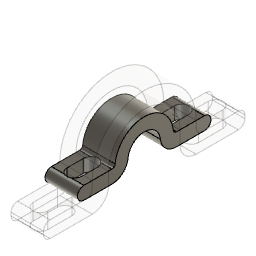
spiral_sleve_holders (Autodesk Fusion 360 design; units mm, degrees)
Autodesk Fusion 360 part; units mm, degrees
sketch "Sketch1" plane through (0, 0, 0) normal (1, 0, 0) x (0, 1, 0) in component "small_spiral_sleve_holder"
  circle A0 centre (0, 0) radius 5
  circle A1 centre (0, 0) radius 9
  line L0 (0, 0) -> (0, -5) construction
  line L1 (8.0623, -4) -> (20.5623, -4)
  line L2 (20.5623, -4) -> (20.5623, 0)
  line L3 (20.5623, 0) -> (9, 0)
  line L4 (-20.5623, 0) -> (-9, 0)
  line L5 (-20.5623, -4) -> (-20.5623, 0)
  line L6 (-8.0623, -4) -> (-20.5623, -4)
  line L7 (-8.0623, -4) -> (8.0623, -4)
  line L8 (-5, 0) -> (-5, -4)
  line L9 (5, 0) -> (5, -4)
  dimension "d1" = 10
  dimension "d2" = 4
  dimension "d57" = 1
  dimension "d58" = 4
  dimension "d59" = 12.5
  constraint coincident A0.centre A1.centre
  constraint coincident A0 L0.end
  constraint vertical L0
  constraint coincident A1 L1.start
  constraint horizontal L1
  constraint perpendicular L1 L2
  constraint perpendicular L2 L3
  constraint coincident A1 L3.end
  constraint symmetric L0 L1.start L6.start
  constraint symmetric L0 L1.end L5.start
  constraint symmetric L0 L2.end L4.start
  constraint symmetric L0 L3.end L4.end
  constraint coincident A0 L8.start
  constraint coincident L7 L8.end
  constraint tangent A0 L8
  constraint perpendicular L7 L8
  constraint coincident A0 L9.start
  constraint coincident L7 L9.end
  constraint tangent A0 L9
  constraint perpendicular L7 L9
  measures "d1" diameter of A0
  measures "d2" distance of A0 A1
  measures "d57" distance of L0.end L1
  measures "d58" distance of L1.end L2.end
  measures "d59" distance of L1.start L1.end
extrude "Extrude1" add sketch "Sketch1" along normal blind 10 contours A0 A1 L7 L8 L9 | A1 L1 L2 L3 | A1 L4 L5 L6 makes body 1 in component "small_spiral_sleve_holder"
sketch "Sketch1 (2)" plane through (0, 0, 0) normal (1, 0, 0) x (0, 1, 0) in component "big_spiral_holder_1"
  circle A0 centre (0, 0) radius 11
  circle A1 centre (0, 0) radius 16
  line L0 (-16, 0) -> (16, 0) construction
  line L1 (-16, 0) -> (-11, 0)
  line L2 (11, 0) -> (16, 0)
  line L3 (-11, 0) -> (-11, -9)
  line L4 (-11, -9) -> (-31, -9)
  line L5 (-31, -9) -> (-31, -4)
  line L6 (-31, -4) -> (-16, -4)
  line L7 (-16, 0) -> (-16, -4)
  line L8 (-11, -9) -> (-6.3246, -9)
  line L9 (0, 0) -> (0, -11) construction
  line L10 (31, -4) -> (16, -4)
  line L11 (31, -9) -> (31, -4)
  line L12 (11, -9) -> (31, -9)
  line L13 (11, 0) -> (11, -9)
  line L14 (16, 0) -> (16, -4)
  line L15 (16, 0) -> (11, 0)
  point P0 (0, -11)
  dimension "d19" = 22
  dimension "d20" = 5
  dimension "d37" = 5
  dimension "d38" = 15
  dimension "d56" = 2
  constraint coincident A0.centre A1.centre
  constraint concentric A0 A1
  constraint coincident A1 L0.start
  constraint coincident A1 L0.end
  constraint horizontal L0
  constraint coincident A0.centre L0
  constraint coincident L0 L1.end
  constraint coincident A0 L1.end
  constraint coincident A0 L2.start
  constraint coincident L0 L2.start
  constraint tangent A0 L3
  constraint perpendicular L3 L4
  constraint perpendicular L4 L5
  constraint perpendicular L5 L6
  constraint coincident A0 L8.end
  constraint parallel L4 L8
  constraint perpendicular L6 L7
  constraint coincident A0 P0
  constraint vertical A0.centre L9.end
  constraint coincident P0 L9.end
  constraint symmetric L0.start L9 L0.end
  constraint symmetric L1.end L9 L2.start
  constraint symmetric L3.end L9 L12.start
  constraint symmetric L4.end L9 L11.start
  constraint symmetric L5.end L9 L10.start
  constraint symmetric L6.end L9 L10.end
  measures "d19" diameter of A0
  measures "d20" distance of A0 A1
  measures "d37" distance of L4 L6
  measures "d38" distance of L5 L7
  measures "d56" distance of L4 P0
extrude "Extrude3" add sketch "Sketch1 (2)" along normal blind 10 separate body contours A0 A1 L1 L2 L15 | A1 L2 L12 L13 L15 | A1 L1 L3 L4 | A1 L10 L11 L12 L14 | A1 L4 L5 L6 L7 makes body 2 in component "big_spiral_holder_1"
sketch "Sketch3" plane through (0, 0, -4) normal (0, 0, 1) x (-1, 0, 0) in component "big_spiral_holder_1"
  line L0 (0, 16) -> (0, 31)
  line L1 (0, 31) -> (-10, 31)
  line L2 (-10, 31) -> (-10, 16)
  line L3 (-10, 16) -> (0, 16)
  line L4 (0, 16) -> (0, -16)
  line L5 (0, 16) -> (-10, 16)
  line L6 (-10, 16) -> (-10, -16)
  line L7 (-2.75, -27) -> (-2.75, -19.5)
  arc A0 (-2.75, -19.5) -> (-7.25, -19.5) centre (-5, -19.5) ccw
  line L8 (-7.25, -19.5) -> (-7.25, -27)
  arc A1 (-7.25, -27) -> (-2.75, -27) centre (-5, -27) ccw
  line L9 (-5, -27) -> (-5, -19.5) construction
  arc A2 (-7.25, 19.5) -> (-2.75, 19.5) centre (-5, 19.5) ccw
  line L10 (-5, 19.5) -> (-5, 27) construction
  line L11 (-2.75, 19.5) -> (-2.75, 27)
  arc A3 (-2.75, 27) -> (-7.25, 27) centre (-5, 27) ccw
  line L12 (-7.25, 27) -> (-7.25, 19.5)
  line L13 (-10, -16) -> (0, -16)
  line L14 (0, -31) -> (0, -16)
  line L15 (0, -16) -> (-10, -16)
  line L16 (-10, -16) -> (-10, -31)
  line L17 (-10, -31) -> (0, -31)
  dimension "d41" = 4.5
  dimension "d42" = 7.5
  dimension "d43" = 4.5
  dimension "d44" = 7.5
  dimension "d45" = 4
  dimension "d46" = 5
  dimension "d47" = 5
  dimension "d48" = 4
  constraint tangent L7 A0
  constraint tangent A0 L8
  constraint parallel L7 L8
  constraint tangent L8 A1
  constraint tangent L7 A1
  constraint parallel L9 L14
  constraint tangent L11 A3
  constraint tangent A3 L12
  constraint parallel L11 L12
  constraint tangent A2 L12
  constraint tangent A2 L11
  measures "d41" diameter of A0
  measures "d42" distance of A1.centre A0.centre
  measures "d43" diameter of A3
  measures "d44" distance of A2.centre L10.end
  measures "d45" distance of A1.centre L17
  measures "d46" distance of L9 L14
  measures "d47" distance of L2 L10
  measures "d48" distance of L1 L10.end
extrude "Extrude4" cut sketch "Sketch3" against normal blind 10 contours L7 A0 L8 A1 | A2 L11 A3 L12 bodies 2 in component "big_spiral_holder_1"
fillet "Fillet1" radius 5 2 edges at (5, -11, -9) (5, 11, -9) on bodies 2 in component "big_spiral_holder_1"
fillet "Fillet1" radius 2 6 edges at (5, -31, -9) (5, -31, -4) (5, -16, -4) (5, 31, -4) (5, 31, -9) (5, 16, -4) on bodies 2 in component "big_spiral_holder_1"
sketch "Sketch3 (2)" plane through (0, 0, 0) normal (0, 0, 1) x (-1, 0, 0) in component "small_spiral_sleve_holder"
  line L0 (0, 9) -> (0, 20.5623)
  line L1 (0, 20.5623) -> (-10, 20.5623)
  line L2 (-10, 20.5623) -> (-10, 9)
  line L3 (-10, 9) -> (0, 9)
  line L4 (0, -20.5623) -> (0, -9)
  line L5 (0, -9) -> (-10, -9)
  line L6 (-10, -9) -> (-10, -20.5623)
  line L7 (-10, -20.5623) -> (0, -20.5623)
  line L8 (-2.75, -16.5623) -> (-2.75, -11.5623)
  arc A0 (-2.75, -11.5623) -> (-7.25, -11.5623) centre (-5, -11.5623) ccw
  line L9 (-7.25, -11.5623) -> (-7.25, -16.5623)
  arc A1 (-7.25, -16.5623) -> (-2.75, -16.5623) centre (-5, -16.5623) ccw
  line L10 (-5, -16.5623) -> (-5, -11.5623) construction
  arc A2 (-2.75, 16.5623) -> (-7.25, 16.5623) centre (-5, 16.5623) ccw
  line L11 (-5, 11.5623) -> (-5, 16.5623) construction
  arc A3 (-7.25, 11.5623) -> (-2.75, 11.5623) centre (-5, 11.5623) ccw
  line L12 (-7.25, 16.5623) -> (-7.25, 11.5623)
  line L13 (-2.75, 11.5623) -> (-2.75, 16.5623)
  circle A4 centre (-21.9949, -14.6483) radius 2
  circle A5 centre (-21.9949, 15.3517) radius 2
  dimension "d60" = 4.5
  dimension "d61" = 5
  dimension "d62" = 4
  dimension "d63" = 4.5
  dimension "d64" = 5
  dimension "d65" = 4
  dimension "d66" = 5
  dimension "d67" = 5
  dimension "d76" = 4
  dimension "d77" = 4
  dimension "d78" = 30
  constraint tangent L8 A0
  constraint tangent A0 L9
  constraint parallel L8 L9
  constraint tangent L9 A1
  constraint tangent L8 A1
  constraint vertical L10
  constraint tangent A2 L13
  constraint tangent A2 L12
  constraint parallel L12 L13
  constraint tangent A3 L12
  constraint tangent A3 L13
  constraint vertical L11
  constraint vertical A4.centre A5.centre
  measures "d60" diameter of A0
  measures "d61" distance of A1.centre A0.centre
  measures "d62" distance of L7 A1.centre
  measures "d63" diameter of A2
  measures "d64" distance of A2.centre L11.start
  measures "d65" distance of L1 A2.centre
  measures "d66" distance of L2 L11
  measures "d67" distance of L4 L10
  measures "d76" diameter of A4
  measures "d77" diameter of A5
  measures "d78" vertical distance of A4.centre A5.centre
extrude "Extrude3'" cut sketch "Sketch3 (2)" against normal blind 10 contours L8 A0 L9 A1 | A2 A3 L12 L13 bodies 1 in component "small_spiral_sleve_holder"
fillet "Fillet2" radius 5 2 edges at (5, 5, -4) (5, -5, -4) on bodies 1 in component "small_spiral_sleve_holder"
fillet "Fillet2" radius 2 4 edges at (5, -20.5623, 0) (5, -20.5623, -4) (5, 20.5623, 0) (5, 20.5623, -4) on bodies 1 in component "small_spiral_sleve_holder"
fillet "Fillet2" radius 1 2 edges at (5, -9, 0) (5, 9, 0) on bodies 1 in component "small_spiral_sleve_holder"
component "small_spiral_sleve_holder" placed x (1, 0, 0) y (0, 1, 0) z (0, 0, 1) at (0, 0, 0)
component "big_spiral_holder_1" placed x (1, 0, 0) y (0, 1, 0) z (0, 0, 1) at (0, 0, 0)
